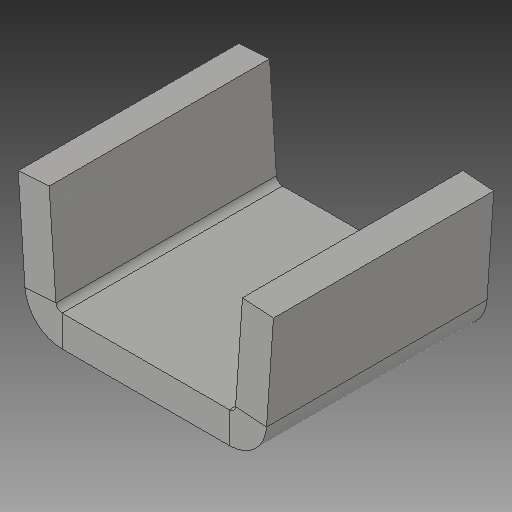
# Autodesk Inventor part: øre
Saved by Autodesk Inventor 2018 (Build 220112000, 112)
## iProperties
Created: 2019-09-25
Part Number: øre
Material: Steel
Document SubType Name: Sheet Metal
Designer: loppen
Density: 7.85 g/cm^3
Sheet Metal Rule: Default_mm
Appearance: Light Gray
Author: loppen
Autodesk Inventor part; units mm, degrees
ref_plane "YZ Plane" through (0, 0, 0) normal (1, 0, 0) x (0, 1, 0)
ref_plane "XZ Plane" through (0, 0, 0) normal (0, 1, 0) x (-1, 0, 0)
ref_plane "XY Plane" through (0, 0, 0) normal (0, 0, 1) x (1, 0, 0)
sketch "Sketch1" plane through (0, 0, 0) normal (0, 1, 0) x (-1, 0, 0)
  line L0 (0, 0) -> (0, -27.002) construction
  line L1 (19.064, 12.0028) -> (-19.064, 12.0028)
  line L2 (-19.064, 12.0028) -> (-19.064, -23.4972)
  line L3 (-19.064, -23.4972) -> (19.064, -23.4972)
  line L4 (19.064, -23.4972) -> (19.064, 12.0028)
  dimension "d0" = 35.5
  dimension "d12" = 38.128
  measures "d0" distance between parallel lines of L1 L3
  measures "d12" distance of L2.end L3.end
extrude "Plate1" add sketch "Sketch1" along normal blind 5
sketch "Sketch2" plane through (-14.0762, 0.3488, 12.0028) normal (-0.9975641, -0.0697565, 0) x (0.0697565, -0.9975641, 0)
  line L0 (0, -35.5) -> (0, 0)
  line L1 (0, 0) -> (-21.37, 0)
  line L2 (-21.37, 0) -> (-21.37, -35.5)
  line L3 (-21.37, -35.5) -> (0, -35.5)
  constraints: 6 end point, 1 horizontal, 1 perpendicular, 1 vertical
edge flange "Flange1" height 21.37 angle 86 thickness 5 bend radius 1 thickness toward (-0.9975641, -0.0697565, 0) relief straight relief width 5 relief depth 2.5 corner gap 1 corner form 0 edges at (-19.064, 5, -5.7472) (19.064, 5, -5.7472) wall of the first edge with corners at (-14.0762, 0.3488, -23.4972) (-14.0762, 0.3488, 12.0028) (-15.5669, 21.6667, 12.0028) (-15.5669, 21.6667, -23.4972)
bend "Bend1"
corner "Corner1"
equation "\"d1\" = Thickness"
equation "\"d2\" = BendReliefWidth"
equation "\"d3\" = BendReliefDepth"
equation "\"d4\" = MinimumRemnant"
equation "\"d5\" = TransitionRadius"
equation "\"d8\" = BendRadius"
equation "\"d9\" = CornerReliefSize"
equation "\"d10\" = GapSize"
equation "\"d11\" = JacobiRadiusSize"
equation "\"BendReliefWidth\" = Thickness"
equation "\"BendReliefDepth\" = 0.5 * Thickness"
equation "\"TransitionRadius\" = BendRadius"
equation "\"JacobiRadiusSize\" = BendRadius"
equation "\"GapSize\" = Thickness"
equation "\"Thickness\" = 5"
equation "\"MinimumRemnant\" = 10"
equation "\"BendRadius\" = 1"
equation "\"CornerReliefSize\" = 20"
body "Solid1"
